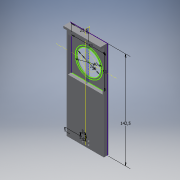
# Autodesk Inventor part: PMT_Adaptor_Shutter
Saved by Autodesk Inventor 2016 (Build 200138000, 138)
## iProperties
Created: 2016-05-11
Part Number: PMT_Adaptor_Shutter
Material: Generic
Document SubType Name: Modeling
Designer: pupa
Density: 1 g/cm^3
Appearance: Default
Author: pupa
Autodesk Inventor part; units mm, degrees
ref_plane "YZ Plane" through (0, 0, 0) normal (1, 0, 0) x (0, 1, 0)
ref_plane "XZ Plane" through (0, 0, 0) normal (0, 1, 0) x (-1, 0, 0)
ref_plane "XY Plane" through (0, 0, 0) normal (0, 0, 1) x (1, 0, 0)
sketch "Shutter" plane through (0, 0, 0) normal (0, 0, 1) x (1, 0, 0)
  line L0 (-25.5, 25.2655) -> (25.5, 25.2655)
  line L1 (25.5, 25.2655) -> (25.5, -25.7345)
  line L2 (25.5, -25.7345) -> (-25.5, -25.7345)
  line L3 (-25.5, -25.7345) -> (-25.5, 25.2655)
  line L4 (0, -25.7345) -> (0, 25.2655) construction
  circle A0 centre (0, -0.2345) radius 11 construction
  circle A1 centre (0, -0.2345) radius 17.5
  circle A2 centre (0, -0.2345) radius 20
  line L5 (-27.3, 37.7655) -> (-27.3, -89.7345)
  circle A3 centre (-4.3962, -99.7345) radius 1.5
  circle A4 centre (-4.3962, -94.7345) radius 1.5
  circle A5 centre (4.3962, -94.7345) radius 1.5
  circle A6 centre (4.3962, -99.7345) radius 1.5
  line L6 (27.3, 37.7655) -> (27.3, -89.7345)
  line L7 (-49, 0) -> (42, 0) construction
  line L8 (-27.3, 37.7655) -> (27.3, 37.7655)
  line L9 (-10, -104.7345) -> (10, -104.7345)
  line L10 (27.3, 37.7655) -> (-27.3, 37.7655)
  line L11 (-27.3, -89.7345) -> (27.3, -89.7345)
  line L12 (-27.3, -86.7345) -> (27.3, -86.7345)
  line L13 (0, -104.7345) -> (-10, -104.7345)
  line L14 (-10, -104.7345) -> (-10, -89.7345)
  line L15 (0, -104.7345) -> (10, -104.7345)
  line L16 (10, -104.7345) -> (10, -89.7345)
  point P0 (0, 17.2655)
  point P1 (0, 10.7655)
  dimension "d0" = 22
  dimension "d1" = 35
  dimension "d2" = 40
  dimension "d12" = 3
  dimension "d13" = 3
  dimension "d14" = 5
  dimension "d16" = 25.5
  dimension "d17" = 51
  dimension "d18" = 51
  dimension "d33" = 142.5
  dimension "d34" = 5
  dimension "d37" = 3
  dimension "d40" = 10
  dimension "d41" = 10
  constraints: 34 end point, 5 centre point, 4 coincident, 4 midpoint, 4 perpendicular, 4 point on line, 3 parallel, 2 vertical alignment, 1 horizontal, 10 other
  measures "d2" diameter of A2
  measures "d12" diameter of A3
  measures "d13" diameter of A4
  measures "d14" distance of A3.centre A4.centre
  measures "d16" distance between parallel lines of L4 L3
  measures "d17" distance between parallel lines of L2 L0
  measures "d18" distance between parallel lines of L1 L3
  measures "d33" distance between parallel lines of L9 L8
  measures "d34" distance from line of A3.centre L9
  measures "d37" distance between parallel lines of L11 L12
  measures "d40" distance of L9.start L13.start
  measures "d41" distance of L9.end L13.start
extrude "Extrusion1" add sketch "Shutter" against normal blind 1.5 contours L0 L1 L2 L3 | A2 | L8 L6 L12 L5 | L12 L6 L11 L5 | L11 L16 L9 L14
extrude "Extrusion2" add sketch "Shutter" along normal blind 5 contours L8 L6 L12 L5 | L12 L6 L11 L5 | L11 L16 L9 L14
ref_plane "Work Plane2" through (0, -85.7345, -1.5) normal (-1, 0, 0) x (0, 0, 1)
sketch "Sketch4" plane through (0, 0, 5) normal (0, 0, 1) x (1, 0, 0)
  line L0 (-27.3, 37.7655) -> (-27.3, -85.7345)
  line L1 (-27.3, 37.7655) -> (-27.3, 34.7655)
  line L2 (-27.3, 34.7655) -> (27.3, 34.7655)
  line L3 (27.3, -85.7345) -> (27.3, 37.7655)
  line L4 (27.3, 37.7655) -> (-27.3, 37.7655)
  line L5 (27.3, 37.7655) -> (-27.3, 37.7655)
  line L6 (-27.3, 34.7655) -> (-27.3, 37.7655)
  line L7 (27.3, 34.7655) -> (27.3, 37.7655)
  line L8 (27.3, -104.7345) -> (-10, -104.7345) projected
  line L9 (-27.3, -89.7345) -> (-27.3, 37.7655) projected
  line L10 (-27.3, -89.7345) -> (27.3, -89.7345)
  line L11 (27.3, 37.7655) -> (27.3, -89.7345) projected
  line L12 (27.3, -86.7345) -> (-27.3, -86.7345)
  line L13 (-27.3, -89.7345) -> (-27.3, -86.7345)
  line L14 (27.3, -89.7345) -> (27.3, -86.7345)
  point P0 (0, 0)
  dimension "d29" = 3
  dimension "d38" = 15
  dimension "d39" = 3
  constraints: 24 end point, 3 point on line, 2 collinear, 2 perpendicular, 3 other
  measures "d29" distance of L0.start L1.end
  measures "d38" vertical distance of L8.end L10.start
  measures "d39" distance between parallel lines of L10 L12
extrude "Extrusion4" add sketch "Sketch4" along normal blind 5 contours L4 L3 L2 L0 | L12 L11 L10 L9
sketch "Sketch5" plane through (-10, -104.7345, -1.5) normal (0, -1, 0) x (1, 0, 0)
  line L0 (0, 6.5) -> (20, 6.5) projected
  circle A0 centre (10, 6.5) radius 2
  dimension "d42" = 4
  constraints: 1 centre point, 1 midpoint
  measures "d42" diameter of A0
extrude "Extrusion5" cut sketch "Sketch5" against normal up to surface (15 mm away)
body "Solid1"
